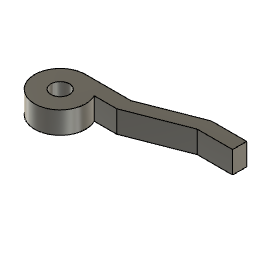
clasp v1 (Autodesk Fusion 360 design; units mm, degrees)
Autodesk Fusion 360 part; units mm, degrees
sketch "Sketch1" plane through (0, 0, 0) normal (0, 0, 1) x (1, 0, 0)
  circle A0 centre (0, 0) radius 0.8344
  line L0 (0, 0) -> (-2.286, 0) construction
  line L1 (0, 2.286) -> (4.064, 2.286)
  line L2 (2.0478, 1.016) -> (4.064, 1.016)
  line L3 (12.446, 4.318) -> (9.271, 4.318)
  line L4 (12.446, 4.318) -> (12.446, 3.048)
  line L5 (12.446, 3.048) -> (9.271, 3.048)
  line L6 (4.064, 2.286) -> (9.271, 4.318)
  line L7 (4.064, 1.016) -> (9.271, 3.048)
  arc A1 (0, 2.286) -> (2.0478, 1.016) centre (0, 0) ccw
  dimension "d1" = 1.6688
  dimension "d2" = 4.572
  dimension "d9" = 3.175
  dimension "d10" = 1.27
  dimension "d11" = 3.175
  constraint coincident A0.centre L0.start
  constraint coincident L0.end A1
  constraint horizontal L0
  constraint perpendicular L3 L4
  constraint perpendicular L4 L5
  constraint parallel L6 L7
  measures "d1" diameter of A0
  measures "d2" diameter of A1
  measures "d9" distance of L3.start L3.end
  measures "d10" distance of L3.start L4.end
  measures "d11" distance of L4.end L5.end
extrude "Extrude1" add sketch "Sketch1" along normal blind 1.9812
